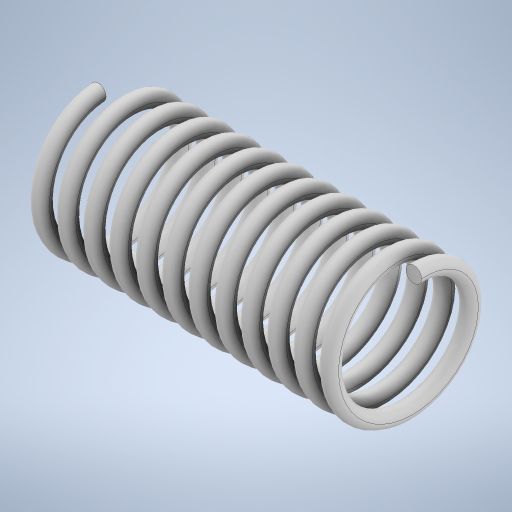
# Autodesk Inventor part: Hudson 1-59
Saved by Autodesk Inventor 2024.2 (Build 282272000, 272)
## iProperties
Created: 2024-10-06
Part Number: Hudson 1-59
Material: Genérico
Document SubType Name: Modeling
Designer: Monica Mora
Density: 1 g/cm^3
Appearance: Valor por defecto
Author: Monica Mora
Autodesk Inventor part; units mm, degrees
ref_plane "YZ Plane" through (0, 0, 0) normal (1, 0, 0) x (0, 1, 0)
ref_plane "XZ Plane" through (0, 0, 0) normal (0, 1, 0) x (-1, 0, 0)
ref_plane "XY Plane" through (0, 0, 0) normal (0, 0, 1) x (1, 0, 0)
sketch "Boceto1" plane through (0, 0, 0) normal (0, 0, 1) x (1, 0, 0)
  line L0 (0, 0) -> (-6.4646, 0)
  circle A0 centre (0, 2) radius 0.25
  dimension "d1" = 0.5
  dimension "d10" = 4
  constraints: 2 end point, 1 centre point, 1 horizontal
  measures "d1" diameter of A0
  measures "d10" diameter of A0.centre L0
coil "Bobina1" sketch "Boceto1" operation add axis through (0, 0, 0) along (-1, 0, 0) pitch 0.8333 turns 12 hand right
